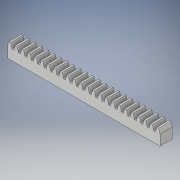
# Autodesk Inventor part: Cremallera
Saved by Autodesk Inventor 2019 (Build 230136000, 136)
## iProperties
Created: 2020-02-02
Part Number: Cremallera
Material: Generic
Document SubType Name: Modeling
Designer: Elías Sánchez
Density: 1 g/cm^3
Appearance: Default
Author: Elías Sánchez
Autodesk Inventor part; units mm, degrees
ref_plane "YZ Plane" through (0, 0, 0) normal (1, 0, 0) x (0, 1, 0)
ref_plane "XZ Plane" through (0, 0, 0) normal (0, 1, 0) x (-1, 0, 0)
ref_plane "XY Plane" through (0, 0, 0) normal (0, 0, 1) x (1, 0, 0)
sketch "Sketch1" plane through (0, 0, 0) normal (0, 0, 1) x (1, 0, 0)
  line L0 (0, 0) -> (148.627, 0)
  line L1 (148.627, 0) -> (148.627, 10)
  line L2 (148.627, 10) -> (0, 10)
  line L3 (0, 10) -> (0, 0)
  dimension "d0" = 148.627
  dimension "d1" = 10
  constraints: 8 end point, 2 parallel, 1 horizontal, 1 perpendicular
  measures "d0" distance of L2.end L1.end
  measures "d1" distance of L0.end L1.end
extrude "Extrusion1" add sketch "Sketch1" along normal blind 12
sketch "Sketch2" plane through (0, 0, 12) normal (0, 0, 1) x (1, 0, 0)
  arc A0 (4.1138, 10) -> (2.9206, 14.6043) centre (-12.3652, 8.1863) ccw
  arc A1 (2.9206, 14.6043) -> (1.1932, 14.6043) centre (2.0569, -7.3787) ccw
  arc A2 (1.1932, 14.6043) -> (0, 10) centre (16.479, 8.1863) ccw
  line L0 (0, 0) -> (148.627, 0) projected
  line L1 (148.627, 0) -> (148.627, 10) projected
  line L2 (148.627, 10) -> (0, 10) projected
  line L3 (0, 10) -> (0, 0) projected
  line L4 (148.627, 10) -> (0, 10) projected
  line L5 (0, 10) -> (4.1138, 10)
  dimension "d4" = 16.5785
  dimension "d5" = 16.5785
  dimension "d6" = 22
  dimension "d7" = 28.8442
  dimension "d8" = 1.1932
  dimension "d9" = 6.418
  dimension "d10" = 4.6043
  dimension "d11" = 1.1932
  constraints: 6 point on circle, 3 centre point, 2 end point, 1 collinear
  measures "d4" radius of A2
  measures "d5" radius of A0
  measures "d6" radius of A1
  measures "d7" distance of A0.centre A2.centre
  measures "d8" horizontal distance of L4.end A2.start
  measures "d9" vertical distance of A1.start A0.centre
  measures "d10" vertical distance of L4.end A2.start
  measures "d11" horizontal distance of L5.end A1.start
extrude "Extrusion2" add sketch "Sketch2" against normal blind 12 contours L2 A2 A1 A0
pattern_linear "Rectangular Pattern1" count 24 spacing 6.2832 along (1, 0, 0) of "Extrusion2"
body "Solid1"
